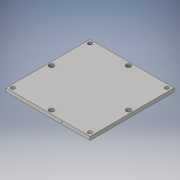
# Autodesk Inventor part: cold_plate
Saved by Autodesk Inventor 2016 (Build 200138000, 138)
## iProperties
Created: 2016-02-26
Part Number: cold_plate
Material: Generic
Document SubType Name: Modeling
Designer: USKHNGO
Density: 1 g/cm^3
Appearance: Default
Author: USKHNGO
Autodesk Inventor part; units mm, degrees
ref_plane "YZ Plane" through (0, 0, 0) normal (1, 0, 0) x (0, 1, 0)
ref_plane "XZ Plane" through (0, 0, 0) normal (0, 1, 0) x (-1, 0, 0)
ref_plane "XY Plane" through (0, 0, 0) normal (0, 0, 1) x (1, 0, 0)
sketch "Sketch1" plane through (0, 0, 0) normal (0, 1, 0) x (-1, 0, 0)
  line L0 (0, 0) -> (-76.2, 0)
  line L1 (-76.2, 0) -> (-76.2, -76.2)
  line L2 (-76.2, -76.2) -> (0, -76.2)
  line L3 (0, -76.2) -> (0, 0)
  line L4 (-38.1, -76.2) -> (-38.1, -73.025)
  circle A0 centre (-38.1, -73.025) radius 2.1844
  line L5 (0, -38.1) -> (-3.175, -38.1)
  line L6 (-38.1, 0) -> (-38.1, -3.175)
  line L7 (-76.2, -38.1) -> (-73.025, -38.1)
  circle A1 centre (-3.175, -38.1) radius 2.1844
  circle A2 centre (-73.025, -38.1) radius 2.1844
  circle A3 centre (-38.1, -3.175) radius 2.1844
  circle A4 centre (-3.175, -73.025) radius 1.778
  circle A5 centre (-3.175, -3.175) radius 1.778
  circle A6 centre (-73.025, -3.175) radius 1.778
  circle A7 centre (-73.025, -73.025) radius 1.778
  dimension "d0" = 76.2
  dimension "d1" = 76.2
  dimension "d2" = 3.175
  dimension "d3" = 4.3688
  dimension "d4" = 3.175
  dimension "d5" = 3.175
  dimension "d6" = 3.175
  dimension "d7" = 4.3688
  dimension "d8" = 4.3688
  dimension "d9" = 4.3688
  dimension "d10" = 3.556
  dimension "d11" = 3.556
  dimension "d12" = 3.556
  dimension "d13" = 3.556
  constraints: 16 end point, 8 centre point, 4 midpoint, 3 horizontal, 2 parallel, 2 vertical, 1 coincident, 1 perpendicular
  measures "d0" distance of L2.end L1.end
  measures "d1" distance of L1.end L0.end
  measures "d2" distance of L4.start L4.end
  measures "d3" diameter of A0
  measures "d4" distance of L5.start L5.end
  measures "d5" distance of L6.start L6.end
  measures "d6" distance of L7.start L7.end
  measures "d7" diameter of A1
  measures "d8" diameter of A2
  measures "d9" diameter of A3
  measures "d10" diameter of A4
  measures "d11" diameter of A5
  measures "d12" diameter of A6
  measures "d13" diameter of A7
extrude "Extrusion1" add sketch "Sketch1" along normal blind 3.302
sketch "Sketch2" plane through (0, 0, 0) normal (0, 0, 1) x (1, 0, 0)
  line L0 (76.2, 0) -> (76.2, 3.302) projected
  circle A0 centre (50.8, 1.651) radius 0.508
  point P0 (0, 0)
  dimension "d17" = 1.016
  constraints: 1 centre point
  measures "d17" diameter of A0
extrude "Extrusion2" cut sketch "Sketch2" against normal blind 12.7
body "Solid1"
